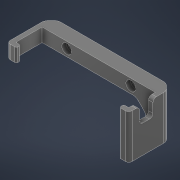
# Autodesk Inventor part: mount_enclosure_coral_dev_board
Saved by Autodesk Inventor 2021 (Build 250183000, 183)
## iProperties
Created: 2021-02-24
Part Number: mount_enclosure_coral_dev_board
Material: ABS Plastic
Document SubType Name: Modeling
Designer: User
Density: 1.06 g/cm^3
Appearance: Smooth - Black
Author: User
Autodesk Inventor part; units mm, degrees
ref_plane "YZ Plane" through (0, 0, 0) normal (1, 0, 0) x (0, 1, 0)
ref_plane "XZ Plane" through (0, 0, 0) normal (0, 1, 0) x (-1, 0, 0)
ref_plane "Work Plane1" through (0, 0, 0) normal (0, 0, 1) x (1, 0, 0)
sketch "base_sketch" plane through (0, 0, 0) normal (0, 0, 1) x (1, 0, 0)
  circle A0 centre (0, -125.6462) radius 1.5 projected
  circle A1 centre (-38, -125.6462) radius 1.5 projected
  line L0 (14.5, -121.6462) -> (-52.5, -121.6462)
  line L1 (-52.5, -121.6462) -> (-52.5, -129.6462)
  line L2 (-52.5, -129.6462) -> (14.5, -129.6462)
  line L3 (14.5, -129.6462) -> (14.5, -121.6462)
  line L4 (-19, -121.6462) -> (-19, -129.6462) construction
  point P0 (0, 0)
  dimension "d1" = 67
  dimension "d4" = 38
  dimension "d5" = 19
  dimension "d6" = 4
  dimension "d7" = 4
  constraints: 10 end point, 2 midpoint, 2 parallel, 1 horizontal, 1 perpendicular
  measures "d1" distance between parallel lines of L1 L3
  measures "d4" distance of A1.centre A0.centre
  measures "d5" distance from line of L4 A0.centre
  measures "d6" distance from line of L0 A0.centre
  measures "d7" distance from line of A0.centre L2
extrude "base" add sketch "base_sketch" along normal blind 8
sketch "holes_bolt_head_sketch" plane through (0, 0, 8) normal (0, 0, 1) x (1, 0, 0)
  circle A0 centre (0, -125.6462) radius 1.5 construction
  circle A1 centre (0, -125.6462) radius 2.9
  circle A2 centre (-38, -125.6462) radius 1.5 construction
  circle A3 centre (-38, -125.6462) radius 2.9
  point P0 (0, 0)
  dimension "d10" = 5.8
  dimension "d11" = 5.8
  constraints: 2 centre point, 2 coincident
  measures "d10" diameter of A3
  measures "d11" diameter of A1
extrude "holes_bolt_head" cut sketch "holes_bolt_head_sketch" against normal blind 3.2
fillet "bolt_head_fillet" radius 0.5 2 edges at (-40.9, -125.6462, 4.8) (-2.9, -125.6462, 4.8)
sketch "walls_sketch" plane through (-52.5, -129.6462, 0) normal (0, -1, 0) x (1, 0, 0)
  line L0 (0, 0) -> (67, 0) projected
  line L1 (67, 0) -> (67, 8) projected
  line L2 (0, 8) -> (67, 8) projected
  line L3 (0, 0) -> (0, 8) projected
  line L4 (67, 8) -> (0, 8) projected
  line L5 (0, 8) -> (0, 23.7)
  line L6 (0, 23.7) -> (3, 23.7)
  line L7 (0, 23.7) -> (3, 23.7) construction
  line L8 (3, 23.7) -> (3, 26.3)
  line L9 (3, 26.3) -> (-2.6, 26.3)
  line L10 (-2.6, 26.3) -> (-2.6, 0)
  line L11 (0, 0) -> (67, 0) projected
  line L12 (-2.6, 0) -> (0, 0)
  line L13 (0, 0) -> (0, 8) projected
  line L14 (33.5, 8) -> (33.5, 0) construction
  line L15 (67, 8) -> (67, 23.7)
  line L16 (67, 23.7) -> (64, 23.7)
  line L17 (64, 23.7) -> (64, 26.3)
  line L18 (64, 26.3) -> (69.6, 26.3)
  line L19 (69.6, 26.3) -> (69.6, 0)
  line L20 (69.6, 0) -> (67, 0)
  line L21 (0, 8) -> (67, 8) projected
  line L22 (61.6, 8) -> (69.6, 8)
  line L23 (69.6, 8) -> (69.6, 0)
  line L24 (69.6, 0) -> (61.6, 0)
  line L25 (61.6, 0) -> (61.6, 8)
  point P0 (52.5, 0)
  dimension "d15" = 15.7
  dimension "d16" = 3
  dimension "d17" = 360
  dimension "d18" = 2.6
  dimension "d19" = 2.6
  dimension "d41" = 8
  constraints: 36 end point, 6 perpendicular, 5 symmetric about line, 3 horizontal, 2 midpoint, 2 parallel, 2 point on line, 1 collinear, 1 vertical
  measures "d15" distance of L2.start L5.end
  measures "d16" distance of L5.end L6.end
  measures "d18" distance between parallel lines of L3 L10
  measures "d19" distance between parallel lines of L9 L6
  measures "d41" distance of L22.start L22.end
extrude "wall" add sketch "walls_sketch" against normal up to surface (8 mm away) contours L12 L10 L9 L8 L6 L5 L3
extrude "wall_offset_top" add sketch "walls_sketch" along normal blind 18 and the other way blind 8 contours L15 L16 L17 L18 L19 L22
extrude "wall_offset_bottom" add sketch "walls_sketch" along normal blind 18 and the other way blind 8 contours L25 L2 L1 L0 | L1 L22 L19 L20
fillet "wall_top" radius 2 2 edges at (-55.1, -125.6462, 26.3) (17.1, -134.6462, 26.3)
fillet "wall_tooth" radius 1 4 edges at (-49.5, -125.6462, 26.3) (-49.5, -125.6462, 23.7) (11.5, -134.6462, 26.3) (11.5, -134.6462, 23.7)
chamfer "wall_bottom" distance 4 angle 45 2 edges at (-55.1, -125.6462, 0) (17.1, -134.6462, 0)
fillet "inside" radius 0.5 2 edges at (-52.5, -125.6462, 8) (-52.5, -125.6462, 23.7)
fillet "bottom" radius 4 4 edges at (-55.1, -125.6462, 4) (-51.1, -125.6462, 0) (17.1, -134.6462, 4) (13.1, -134.6462, 0)
chamfer "wall_offset_outside" distance 2 angle 45 1 edges at (9.1, -147.6462, 4)
chamfer "l_corner" distance 6 angle 45 1 edges at (9.1, -129.6462, 4)
fillet "wall_offset_rounding" radius 4 4 edges at (11.1, -147.6462, 4) (9.1, -145.6462, 4) (9.1, -135.6462, 4) (3.1, -129.6462, 4)
sketch "hole_usb_c_sketch" plane through (17.1, -147.6462, 24.3) normal (1, 0, 0) x (0, 0, -1)
  line L0 (0, 26) -> (18.6431, 26) projected
  line L1 (4.37, 26) -> (12.332, 26)
  line L2 (12.332, 26) -> (12.332, 16.5)
  line L3 (12.332, 16.5) -> (4.37, 16.5)
  line L4 (4.37, 16.5) -> (4.37, 26)
  line L5 (24.3, 0.3593) -> (24.3, 26) projected
  point P0 (24.3, 147.6462)
  dimension "d64" = 9.5
  dimension "d65" = 7.962
  dimension "d66" = 11.968
  constraints: 8 end point, 2 parallel, 1 horizontal, 1 perpendicular, 1 point on line
  measures "d64" distance of L3.end L1.start
  measures "d65" distance of L2.end L3.end
  measures "d66" distance between parallel lines of L5 L2
extrude "hole_usb_c" cut sketch "hole_usb_c_sketch" against normal up to surface (2.6 mm away)
fillet "hole_usb_c_rounded" radius 2 4 edges at (15.8, -131.1462, 19.93) (15.8, -131.1462, 11.968) (15.8, -121.6462, 19.93) (15.8, -121.6462, 11.968)
equation "\"d5\" = 0.5 * d4"
equation "\"d7\" = d6"
equation "\"d10\" = d11"
body "Solid1"
